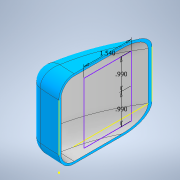
# Autodesk Inventor part: WindShieldGBR
Saved by Autodesk Inventor 2020.1 (Build 241239000, 239)
## iProperties
Created: 2020-03-02
Part Number: WindShieldGBR
Material: Generic
Document SubType Name: Modeling
Designer: super
Density: 1 g/cm^3
Appearance: Default
Author: super
Autodesk Inventor part; units mm, degrees
ref_plane "YZ Plane" through (0, 0, 0) normal (1, 0, 0) x (0, 1, 0)
ref_plane "XZ Plane" through (0, 0, 0) normal (0, 1, 0) x (-1, 0, 0)
ref_plane "XY Plane" through (0, 0, 0) normal (0, 0, 1) x (1, 0, 0)
sketch "Sketch1" plane through (0, 0, 0) normal (0, 1, 0) x (-1, 0, 0)
  line L0 (0, 0) -> (0, -77.216)
  line L1 (0, 0) -> (16.256, 0) construction
  arc A0 (0, -77.216) -> (25.4, -12.446) centre (-125.434846, 9.339528) ccw
  arc A1 (25.4, -12.446) -> (16.442713, -0.893177) centre (15.344344, -10.993631) ccw
  arc A2 (16.442713, -0.893177) -> (0, 0) centre (-0.032832, -152.399996) ccw
  dimension "d0" = 77.216
  dimension "d4" = 16.256
  dimension "d5" = 152.4
  dimension "d6" = 10.16
  dimension "d7" = 152.4
  constraints: 6 point on circle, 4 end point, 3 centre point, 2 tangent, 1 horizontal, 1 vertical
  measures "d0" distance of L0.start L0.end
  measures "d4" distance of L0.start L1.end
  measures "d5" radius of A0
  measures "d6" radius of A1
  measures "d7" radius of A2
extrude "Extrusion1" add sketch "Sketch1" along normal blind 64.77
fillet "Fillet1" radius 12.7 6 edges at (-23.3737, 64.77, -4.7682) (-8.2334, 64.77, -0.2243) (-16.4455, 64.77, -46.2998) (-23.3737, 0, -4.7682) (-8.2334, 0, -0.2243) (-16.4455, 0, -46.2998)
shell "Shell1" thickness 1.778 removed faces 1 at (0, 21.59, -39.006653)
sketch "Sketch2" plane through (0, 0, -12.7) normal (1, 0, 0) x (0, 0, -1)
  line L0 (64.516, 12.7) -> (64.516, 52.07)
  line L1 (-12.7, 12.7) -> (-12.7, 52.07)
  line L2 (47.244, 32.385) -> (47.244, 7.239)
  line L3 (47.244, 32.385) -> (47.244, 57.531)
  line L4 (47.244, 57.531) -> (8.128, 57.531)
  line L5 (8.128, 57.531) -> (8.128, 7.239)
  line L6 (8.128, 7.239) -> (47.244, 7.239)
  line L7 (-0.508165, 12.7) -> (61.34564, 12.7)
  point P0 (-12.7, 0)
  dimension "d13" = 25.146
  dimension "d14" = 25.146
  dimension "d15" = 39.116
  constraints: 10 end point, 2 perpendicular, 2 vertical, 1 parallel
  measures "d13" distance of L2.start L2.end
  measures "d14" distance of L2.start L3.end
  measures "d15" distance of L3.end L4.end
body "Solid1"
